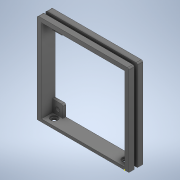
# Autodesk Inventor part: КрепежКулера
Saved by Autodesk Inventor 2020 (Build 240168000, 168)
## iProperties
Created: 2020-04-05
Part Number: КрепежКулера
Material: Типовые
Document SubType Name: Modeling
Designer: Михаил
Density: 1 g/cm^3
Appearance: По умолчанию
Author: Михаил
Autodesk Inventor part; units mm, degrees
ref_plane "YZ Plane" through (0, 0, 0) normal (1, 0, 0) x (0, 1, 0)
ref_plane "XZ Plane" through (0, 0, 0) normal (0, 1, 0) x (-1, 0, 0)
ref_plane "XY Plane" through (0, 0, 0) normal (0, 0, 1) x (1, 0, 0)
sketch "Эскиз1" plane through (0, 0, 0) normal (0, 1, 0) x (-1, 0, 0)
  line L0 (0, 0) -> (120, 0)
  line L1 (120, 0) -> (120, -20)
  line L2 (120, -20) -> (0, -20)
  line L3 (0, -20) -> (0, 0)
  dimension "d0" = 20
  dimension "d1" = 120
  constraints: 8 end point, 2 parallel, 1 horizontal, 1 perpendicular
  measures "d0" distance of L0.end L1.end
  measures "d1" distance of L1.end L2.end
sketch "Эскиз2" plane through (0, 0, 0) normal (0, 1, 0) x (-1, 0, 0)
  line L0 (0, -20) -> (15, -20)
  line L1 (15, -20) -> (15, -16)
  line L2 (15, -16) -> (0, -16)
  line L3 (0, -16) -> (0, -20)
  line L4 (120, -20) -> (105, -20)
  line L5 (105, -20) -> (105, -16)
  line L6 (105, -16) -> (120, -16)
  line L7 (120, -16) -> (120, -20)
  point P0 (0, 0)
  dimension "d2" = 15
  dimension "d3" = 4
  dimension "d39" = 15
  dimension "d40" = 90
  dimension "d41" = 16
  dimension "d42" = 4
  dimension "d43" = 15
  dimension "d44" = 16
  constraints: 16 end point, 4 parallel, 2 horizontal, 2 perpendicular
  measures "d2" distance of L2.end L1.end
  measures "d3" distance of L1.end L0.end
  measures "d39" distance of L5.end L6.end
  measures "d40" distance from line of L0.end L5
  measures "d41" distance from line of point (0, 0) L6
  measures "d42" distance between parallel lines of L4 L6
  measures "d43" distance from line of point (0, 0) L1
  measures "d44" distance from line of point (0, 0) L2
extrude "Выдавливание1" add sketch "Эскиз1" along normal blind 4
sketch "Эскиз3" plane through (0, 4, 0) normal (0, 1, 0) x (1, 0, 0)
  circle A0 centre (-111.5, 10) radius 3.05
  line L0 (-120, 0) -> (0, 0) projected
  line L1 (-120, 20) -> (-120, 0) projected
  circle A1 centre (-8.5, 10) radius 3.05
  line L2 (0, 0) -> (0, 20) projected
  point P0 (0, 16)
  dimension "d9" = 6.1
  dimension "d14" = 10
  dimension "d27" = 8.5
  dimension "d28" = 6.1
  dimension "d29" = 8.5
  dimension "d30" = 10
  constraints: 2 centre point
  measures "d9" diameter of A0
  measures "d14" distance from line of L0 A0.centre
  measures "d27" distance from line of L1 A0.centre
  measures "d28" diameter of A1
  measures "d29" distance from line of L2 A1.centre
  measures "d30" distance from line of L0 A1.centre
sketch "Эскиз4" plane through (0, 4, 0) normal (0, 1, 0) x (1, 0, 0)
  circle A0 centre (-8.5, 10) radius 5.1
  line L0 (-120, 0) -> (0, 0) projected
  line L1 (0, 0) -> (0, 20) projected
  circle A1 centre (-111.5, 10) radius 5.1
  line L2 (-120, 20) -> (-120, 0) projected
  point P0 (0, 16)
  dimension "d11" = 10.2
  dimension "d12" = 10
  dimension "d33" = 8.5
  dimension "d34" = 10.2
  dimension "d35" = 8.5
  dimension "d36" = 10
  constraints: 2 centre point
  measures "d11" diameter of A0
  measures "d12" distance from line of L0 A0.centre
  measures "d33" distance from line of L1 A0.centre
  measures "d34" diameter of A1
  measures "d35" distance from line of L2 A1.centre
  measures "d36" distance from line of L0 A1.centre
extrude "Выдавливание6" cut sketch "Эскиз3" against normal blind 10
extrude "Выдавливание7" cut sketch "Эскиз4" against normal blind 2.4
extrude "Выдавливание8" add sketch "Эскиз2" along normal blind 21
sketch "Эскиз6" plane through (-120, 4, -16) normal (0, 0, 1) x (1, 0, 0)
  circle A0 centre (7.5, 7.5) radius 3.05
  circle A1 centre (112.5, 7.5) radius 3.05
  line L0 (0, 0) -> (120, 0) projected
  line L1 (0, 0) -> (0, 17) projected
  line L2 (105, 0) -> (105, 17) projected
  line L3 (120, 0) -> (120, 17) projected
  point P0 (120, -4)
  point P1 (0, 15)
  point P2 (105, 15)
  point P3 (120, 15)
  dimension "d48" = 6.1
  dimension "d49" = 6.1
  dimension "d50" = 7.5
  dimension "d51" = 7.5
  dimension "d53" = 7.5
  dimension "d66" = 7.5
  constraints: 2 centre point
  measures "d48" diameter of A0
  measures "d49" diameter of A1
  measures "d50" distance from line of L0 A0.centre
  measures "d51" distance from line of L1 A0.centre
  measures "d53" distance from line of L0 A1.centre
  measures "d66" distance from line of L3 A1.centre
sketch "Эскиз7" plane through (-17, 4, -20) normal (0, 0, 1) x (1, 0, 0)
  circle A0 centre (9.5, 7.5) radius 5.1
  circle A1 centre (-95.5, 7.5) radius 5.1
  line L0 (-103, 0) -> (17, 0) projected
  line L1 (-88, 0) -> (-88, 17) projected
  line L2 (17, 0) -> (17, 17) projected
  line L3 (-103, -4) -> (-103, 17) projected
  point P0 (17, -4)
  point P1 (-88, 15)
  point P2 (17, 15)
  point P3 (-103, 15)
  dimension "d54" = 10.2
  dimension "d55" = 10.2
  dimension "d56" = 7.5
  dimension "d58" = 7.5
  dimension "d59" = 7.5
  dimension "d67" = 7.5
  constraints: 2 centre point
  measures "d54" diameter of A0
  measures "d55" diameter of A1
  measures "d56" distance from line of L0 A1.centre
  measures "d58" distance from line of L2 A0.centre
  measures "d59" distance from line of L0 A0.centre
  measures "d67" distance from line of L3 A1.centre
extrude "Выдавливание9" cut sketch "Эскиз6" against normal blind 21
fillet "Сопряжение4" radius 1 1 edges at (-116.6, 1.6, -10)
sketch "Эскиз8" plane through (-120, 0, 0) normal (0, 0, 1) x (1, 0, 0)
  point P0 (120, 0)
sketch "Эскиз9" plane through (0, 0, 0) normal (0, -1, 0) x (1, 0, 0)
  line L0 (-120, 0) -> (0, 0) projected
  line L1 (0, 0) -> (6, 0)
  line L2 (6, 0) -> (6, -20)
  line L3 (6, -20) -> (0, -20)
  line L4 (0, -20) -> (0, 0)
  line L5 (-120, 0) -> (-126, 0)
  line L6 (-126, 0) -> (-126, -20)
  line L7 (-126, -20) -> (-120, -20)
  line L8 (-120, -20) -> (-120, 0)
  dimension "d68" = 6
  dimension "d69" = 6
  dimension "d70" = 20
  dimension "d71" = 120
  dimension "d72" = 20
  constraints: 16 end point, 4 parallel, 2 horizontal, 2 perpendicular, 1 point on line
  measures "d68" distance of L2.end L3.end
  measures "d69" distance of L7.end L6.end
  measures "d70" distance of L6.end L5.end
  measures "d71" distance between parallel lines of L4 L8
  measures "d72" distance between parallel lines of L0 L3
extrude "Выдавливание11" add sketch "Эскиз9" against normal blind 124
sketch "Эскиз10" plane through (0, 124, 0) normal (0, 1, 0) x (1, 0, 0)
  line L0 (6, 0) -> (6, 20) projected
  line L1 (-126, 20) -> (6, 20) projected
  line L2 (6, 0) -> (-126, 0)
  line L3 (-126, 0) -> (-126, 20)
  line L4 (-126, 20) -> (6, 20)
  line L5 (6, 20) -> (6, 0)
  point P0 (0, 0)
  constraints: 8 end point, 2 parallel, 1 horizontal, 1 perpendicular
extrude "Выдавливание12" add sketch "Эскиз10" along normal blind 6
sketch "Эскиз11" plane through (-126, 0, -20) normal (-1, 0, 0) x (0, 0, 1)
  line L0 (0, 0) -> (20, 0) projected
  line L1 (0, 130) -> (20, 130) projected
  line L2 (7.75, 0) -> (12.25, 0)
  line L3 (12.25, 0) -> (12.25, 130)
  line L4 (12.25, 130) -> (7.75, 130)
  line L5 (7.75, 130) -> (7.75, 0)
  line L6 (20, 0) -> (20, 130) projected
  dimension "d77" = 4.5
  dimension "d78" = 7.75
  constraints: 8 end point, 2 parallel, 2 point on line, 1 horizontal, 1 perpendicular
  measures "d77" distance of L4.end L3.end
  measures "d78" distance between parallel lines of L3 L6
sketch "Эскиз12" plane through (6, 0, 0) normal (1, 0, 0) x (0, 0, -1)
  line L0 (20, 0) -> (0, 0) projected
  line L1 (20, 130) -> (0, 130) projected
  line L2 (7.75, 0) -> (12.25, 0)
  line L3 (12.25, 0) -> (12.25, 130)
  line L4 (12.25, 130) -> (7.75, 130)
  line L5 (7.75, 130) -> (7.75, 0)
  line L6 (20, 0) -> (20, 130) projected
  dimension "d79" = 4.5
  dimension "d80" = 7.75
  constraints: 8 end point, 2 parallel, 2 point on line, 1 horizontal, 1 perpendicular
  measures "d79" distance of L4.end L3.end
  measures "d80" distance between parallel lines of L6 L3
extrude "Выдавливание13" cut sketch "Эскиз11" against normal blind 4.5 contours L5 L1 L3 L0
extrude "Выдавливание14" cut sketch "Эскиз12" against normal blind 4.5 contours L0 L5 L1 L3
sketch "Эскиз13" plane through (0, 130, 0) normal (0, 1, 0) x (1, 0, 0)
  line L0 (-121.5, 12.25) -> (-121.5, 7.75) projected
  line L1 (1.5, 7.75) -> (1.5, 12.25) projected
  line L2 (-121.5, 7.75) -> (1.5, 7.75)
  line L3 (1.5, 7.75) -> (1.5, 12.25)
  line L4 (1.5, 12.25) -> (-121.5, 12.25)
  line L5 (-121.5, 12.25) -> (-121.5, 7.75)
  point P0 (0, 0)
  constraints: 8 end point, 2 parallel, 1 horizontal, 1 perpendicular
extrude "Выдавливание15" cut sketch "Эскиз13" against normal blind 4.5
sketch "Эскиз15" plane through (0, 124, 0) normal (0, -1, 0) x (1, 0, 0)
  line L0 (0, -20) -> (-120, -20) projected
  line L1 (-120, -20) -> (-105, -20)
  line L2 (-105, -20) -> (-105, -16)
  line L3 (-105, -16) -> (-120, -16)
  line L4 (-120, -16) -> (-120, -20)
  line L5 (0, -20) -> (-15, -20)
  line L6 (-15, -20) -> (-15, -16)
  line L7 (-15, -16) -> (0, -16)
  line L8 (0, -16) -> (0, -20)
  point P0 (0, 0)
  dimension "d87" = 15
  dimension "d88" = 4
  dimension "d89" = 15
  dimension "d90" = 4
  constraints: 16 end point, 4 parallel, 2 horizontal, 2 perpendicular
  measures "d87" distance of L3.end L2.end
  measures "d88" distance of L2.end L1.end
  measures "d89" distance of L6.end L7.end
  measures "d90" distance of L5.end L6.end
extrude "Выдавливание16" add sketch "Эскиз15" along normal blind 17
sketch "Эскиз16" plane through (-120, 124, -16) normal (0, 0, 1) x (1, 0, 0)
  circle A0 centre (7.5, -7.5) radius 3.05
  circle A1 centre (112.5, -7.5) radius 3.05
  line L0 (0, -17) -> (0, 0) projected
  line L1 (0, 0) -> (15, 0) projected
  line L2 (105, 0) -> (120, 0) projected
  line L3 (120, 0) -> (120, -17) projected
  point P0 (120, -124)
  dimension "d93" = 6.1
  dimension "d94" = 6.1
  dimension "d95" = 7.5
  dimension "d96" = 7.5
  dimension "d97" = 7.5
  dimension "d98" = 7.5
  constraints: 2 centre point
  measures "d93" diameter of A0
  measures "d94" diameter of A1
  measures "d95" distance from line of L0 A0.centre
  measures "d96" distance from line of L1 A0.centre
  measures "d97" distance from line of L2 A1.centre
  measures "d98" distance from line of L3 A1.centre
extrude "Выдавливание17" cut sketch "Эскиз16" against normal blind 17
sketch "Эскиз17" plane through (6, 0, -20) normal (0, 0, -1) x (-1, 0, 0)
  circle A0 centre (13.5, 116.5) radius 5.1
  circle A1 centre (118.5, 116.5) radius 3.05 projected
  circle A2 centre (118.5, 116.5) radius 5.1
  line L0 (21, 124) -> (21, 107) projected
  line L1 (21, 124) -> (111, 124) projected
  line L2 (111, 124) -> (111, 107) projected
  point P0 (6, 0)
  dimension "d101" = 10.2
  dimension "d102" = 10.2
  dimension "d103" = 7.5
  dimension "d104" = 7.5
  dimension "d105" = 7.5
  dimension "d106" = 7.5
  constraints: 2 centre point, 1 coincident
  measures "d101" diameter of A0
  measures "d102" diameter of A2
  measures "d103" distance from line of L0 A0.centre
  measures "d104" distance from line of L1 A0.centre
  measures "d105" distance from line of L1 A2.centre
  measures "d106" distance from line of L2 A2.centre
fillet "Сопряжение9" radius 2 8 edges at (-105, 107, -18) (-105, 21, -18) (-15, 107, -18) (-15, 21, -18) (6, 130, -3.875) (6, 130, -16.125) (-126, 130, -3.875) (-126, 130, -16.125)
